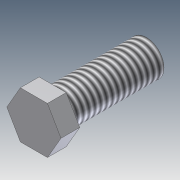
# Autodesk Inventor part: HW-00043
Saved by Autodesk Inventor 2012 (Build 160160000, 160)
## iProperties
Created: 2008-06-03
Part Number: HW-00043
Document SubType Name: Modeling
Designer: mcyr
Density: 1 g/cm^3
Description: Hex head bolt 3/8-16 x 1.250"
Mass: 2.51948 g
Surface Area: 12.6291 cm^2
Volume: 2.51948 cm^3
Material: Default
Title: HW-00012
Author: mcyr
Autodesk Inventor part; units mm, degrees
ref_plane "YZ Plane" through (0, 0, 0) normal (1, 0, 0) x (0, 1, 0)
ref_plane "XZ Plane" through (0, 0, 0) normal (0, 1, 0) x (-1, 0, 0)
ref_plane "XY Plane" through (0, 0, 0) normal (0, 0, 1) x (1, 0, 0)
sketch "Sketch1" plane through (0, 0, 0) normal (0, 0, 1) x (1, 0, 0)
  circle A0 centre (-0.6115, -1.5992) radius 4.7625
  line L0 (-7.9438, -1.5992) -> (-4.2777, 4.7508)
  line L1 (-4.2777, 4.7508) -> (3.0547, 4.7508)
  line L2 (3.0547, 4.7508) -> (6.7209, -1.5992)
  line L3 (6.7209, -1.5992) -> (3.0547, -7.9492)
  line L4 (3.0547, -7.9492) -> (-4.2777, -7.9492)
  line L5 (-4.2777, -7.9492) -> (-7.9438, -1.5992)
  dimension "d10" = 12.7
  dimension "d20" = 9.525
  constraints: 12 end point, 1 centre point, 13 other
  measures "d10" distance between parallel lines of L4 L1
  measures "d20" diameter of A0
extrude "Extrusion1" add sketch "Sketch1" against normal blind 25.4 contours A0
extrude "Extrusion2" add sketch "Sketch1" along normal blind 5.08 contours A0 | L0 L1 L2 L3 L4 L5
thread "Thread2" size "3/8-16 UNC" class "2A" standard "ANSI Unified Screw Threads" full length
body "Solid1"
